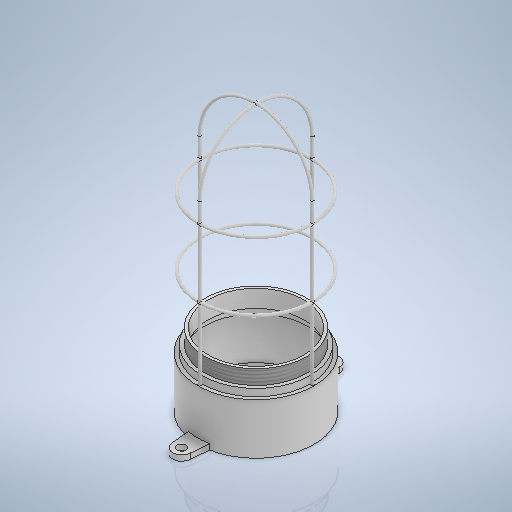
# Autodesk Inventor part: base
Saved by Autodesk Inventor 2025.2 (Build 292293000, 293)
## iProperties
Created: 2025-09-04
Part Number: base
Material: Generic
Document SubType Name: Modeling
Designer: User
Density: 1 g/cm^3
Appearance: Default
Author: User
Autodesk Inventor part; units mm, degrees
ref_plane "YZ Plane" through (0, 0, 0) normal (1, 0, 0) x (0, 1, 0)
ref_plane "XZ Plane" through (0, 0, 0) normal (0, 1, 0) x (-1, 0, 0)
ref_plane "XY Plane" through (0, 0, 0) normal (0, 0, 1) x (1, 0, 0)
sketch "Sketch1" plane through (0, 0, 0) normal (0, 1, 0) x (-1, 0, 0)
  circle A0 centre (0, 0) radius 50.8
  dimension "d0" = 101.6
  constraints: 1 centre point, 1 coincident
  measures "d0" diameter of A0
extrude "Extrusion1" add sketch "Sketch1" along normal blind 44.45
sketch "Sketch2" plane through (0, 44.45, 0) normal (0, 1, 0) x (1, 0, 0)
  circle A0 centre (0, 0) radius 47.625
  dimension "d3" = 95.25
  constraints: 1 centre point, 1 coincident
  measures "d3" diameter of A0
extrude "Extrusion2" add sketch "Sketch2" along normal blind 6.35
sketch "Sketch3" plane through (0, 50.8, 0) normal (0, 1, 0) x (1, 0, 0)
  circle A0 centre (0, 0) radius 44.45
  dimension "d6" = 88.9
  constraints: 1 centre point, 1 coincident
  measures "d6" diameter of A0
extrude "Extrusion3" add sketch "Sketch3" along normal blind 12.7
thread "Thread2"
shell "Shell1" thickness 2.54 removed faces 1 at (5.659463, 63.5, 0)
sketch "Sketch4" plane through (0, 0, 0) normal (0, -1, 0) x (1, 0, 0)
  circle A0 centre (0, -65.0875) radius 3.96875
  arc A1 (-7.9375, -65.0875) -> (7.9375, -65.0875) centre (0, -65.0875) ccw
  line L0 (7.9375, -65.0875) -> (9.338717, -49.903898)
  line L1 (-7.9375, -65.0875) -> (-9.338717, -49.903898)
  arc A2 (-9.338717, -49.903898) -> (9.338717, -49.903898) centre (0, 0) ccw
  circle A3 centre (0, 65.0875) radius 3.96875
  arc A4 (7.9375, 65.0875) -> (-7.9375, 65.0875) centre (0, 65.0875) ccw
  line L2 (7.9375, 65.0875) -> (9.338717, 49.903898)
  line L3 (-7.9375, 65.0875) -> (-9.338717, 49.903898)
  arc A5 (9.338717, 49.903898) -> (-9.338717, 49.903898) centre (0, 0) ccw
  dimension "d16" = 7.9375
  dimension "d17" = 3.96875
  constraints: 8 end point, 8 point on circle, 6 centre point, 3 coincident
  measures "d16" diameter of A0
  measures "d17" radial gap between concentric circles of A1 A0
extrude "Extrusion5" add sketch "Sketch4" against normal blind 4.7625
sketch "Sketch8" plane through (0, 0, 0) normal (1, 0, 0) x (0, 1, 0)
  line L0 (44.45, -50.8) -> (44.45, 50.8)
  line L1 (63.5, -44.45) -> (63.5, 44.45)
  line L2 (44.45, 49.314063) -> (184.15, 49.314063)
  arc A0 (184.15, -49.314063) -> (184.15, 49.314063) centre (184.15, 0) ccw
  line L3 (44.45, -49.314063) -> (184.15, -49.314063)
  point P0 (0, 0)
  constraints: 5 end point, 2 point on circle, 1 centre point, 1 perpendicular, 1 point on line
ref_plane "Work Plane5" through (0, 44.45, 49.314063) normal (0, 1, 0) x (-1, 0, 0)
sketch "Sketch9" plane through (0, 44.45, 49.314063) normal (0, 1, 0) x (-1, 0, 0)
  circle A0 centre (0, 0) radius 1.27
  point P0 (0, -49.314063)
  dimension "d33" = 2.54
  constraints: 1 centre point
  measures "d33" diameter of A0
sweep "Sweep3" add profiles "Sketch9" path "Sketch8" path curves L2 A0 L3
sketch "Sketch10" plane through (0, 0, 0) normal (0, 0, 1) x (1, 0, 0)
  line L0 (-49.365633, 44.992709) -> (-49.365633, 184.692709)
  arc A0 (49.262493, 184.692709) -> (-49.365633, 184.692709) centre (-0.05157, 184.692709) ccw
  line L1 (49.262493, 44.992709) -> (49.262493, 184.692709)
  line L2 (-45.085, 41.91) -> (45.085, 41.91)
  line L3 (1.27, 233.464063) -> (1.27, 184.15)
  point P0 (0, 0)
  constraints: 4 end point, 2 point on circle, 1 centre point
ref_plane "Work Plane6" through (-49.365633, 44.992709, 0) normal (0, 1, 0) x (-1, 0, 0)
sketch "Sketch11" plane through (-49.365633, 44.992709, 0) normal (0, 1, 0) x (-1, 0, 0)
  circle A0 centre (0, 0) radius 1.27
  point P0 (-49.365633, 0)
  dimension "d30" = 2.54
  constraints: 1 centre point
  measures "d30" diameter of A0
sweep "Sweep4" add profiles "Sketch11" path "Sketch10" path curves L0 A0 L1
sketch "Sketch13" plane through (0, 0, 0) normal (0, 0, 1) x (1, 0, 0)
  line L0 (47.992493, 184.692709) -> (47.992493, 44.992709)
  line L1 (0, 0) -> (0, 257.47982)
  circle A0 centre (49.262493, 166.822904) radius 1.27
  line L2 (50.532493, 184.692709) -> (50.532493, 44.992709)
  dimension "d36" = 2.54
  constraints: 2 end point, 1 centre point, 1 tangent, 1 vertical
  measures "d36" diameter of A0
revolve "Revolution2" add sketch "Sketch13" angle 360 about axis through (0, 0, 0) along (0, 1, 0)
sketch "Sketch14" plane through (0, 0, 0) normal (0, 0, 1) x (1, 0, 0)
  circle A0 centre (49.262493, 107.276828) radius 1.27
  line L0 (50.532493, 166.822904) -> (50.532493, 44.992709)
  line L1 (0, -15.543159) -> (0, 212.181328)
  line L2 (1.27, 184.15) -> (1.27, 44.45)
  point P0 (0, 0)
  dimension "d38" = 2.54
  constraints: 2 end point, 1 centre point, 1 parallel, 1 tangent
  measures "d38" diameter of A0
revolve "Revolution3" add sketch "Sketch14" angle 360 about axis through (0, -15.543159, 0) along (0, 1, 0)
body "Solid1"
